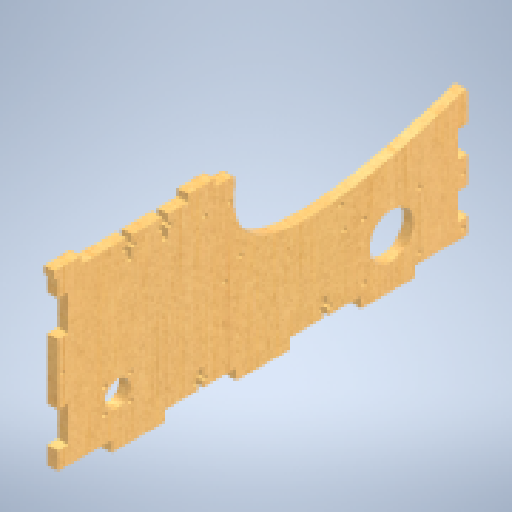
# Autodesk Inventor part: бок
Saved by Autodesk Inventor 2024.2 (Build 282272000, 272)
## iProperties
Created: 2026-01-28
Part Number: бок
Material: Типовые
Document SubType Name: Modeling
Designer: Zakhar
Density: 1 g/cm^3
Appearance: Желтая сосна — массив — светлое морение — со слабым глянцем
Mass: 99.4339 g
Surface Area: 393.183 cm^2
Volume: 99.4339 cm^3
Author: Zakhar
Autodesk Inventor part; units mm, degrees
ref_plane "YZ Plane" through (0, 0, 0) normal (1, 0, 0) x (0, 1, 0)
ref_plane "XZ Plane" through (0, 0, 0) normal (0, 1, 0) x (-1, 0, 0)
ref_plane "XY Plane" through (0, 0, 0) normal (0, 0, 1) x (1, 0, 0)
sketch "Эскиз1" plane through (0, 0, 0) normal (1, 0, 0) x (0, 1, 0)
  line L0 (35.7991, 182.7989) -> (-64.2009, 182.7989)
  line L1 (-64.2009, 182.7989) -> (-64.2009, -47.2011)
  line L2 (-64.2009, -47.2011) -> (35.7991, -47.2011)
  line L3 (35.7991, -47.2011) -> (35.7991, 182.7989)
  spline S0 degree 3 poles (35.7991, 82.7989) (-39.4152, 98.2826) (5.5477, -37.1054) (35.7991, -102.9099) knots 0 0 0 0 1 1 1 1
  line L4 (-4.2009, -47.2011) -> (-19.2009, -47.2011)
  line L5 (-19.2009, -47.2011) -> (-19.2009, -41.2011)
  line L6 (-19.2009, -41.2011) -> (-4.2009, -41.2011)
  line L7 (-4.2009, -41.2011) -> (-4.2009, -47.2011)
  line L8 (-34.2009, -47.2011) -> (-49.2009, -47.2011)
  line L9 (-49.2009, -47.2011) -> (-49.2009, -41.2011)
  line L10 (-49.2009, -41.2011) -> (-34.2009, -41.2011)
  line L11 (-34.2009, -41.2011) -> (-34.2009, -47.2011)
  point P0 (0, 0)
  point P1 (0.0412, 70.0052)
  point P2 (13.562, -47.2011)
  point P3 (-4.2009, -44.2011)
  point P4 (-19.2009, -44.2011)
  point P5 (-34.2009, -44.2011)
  point P6 (-49.2009, -44.2011)
  dimension "d0" = 230
  dimension "d1" = 100
  dimension "d20" = 100
  dimension "d155" = 15
  dimension "d156" = 15
  dimension "d157" = 6
  dimension "d158" = 15
  dimension "d159" = 15
  constraints: 24 end point, 6 parallel, 5 point on line, 4 midpoint, 3 horizontal, 3 perpendicular, 4 other
  measures "d0" distance of L0.end L1.end
  measures "d1" distance of L0.start L0.end
  measures "d20" distance from line of L0 point (35.799, 82.799)
  measures "d155" distance of point (-4.201, -44.201) point (-19.201, -44.201)
  measures "d156" distance of point (-34.201, -44.201) point (-49.201, -44.201)
  measures "d157" distance between parallel lines of L8 L10
  measures "d158" distance of point (-34.201, -44.201) point (-19.201, -44.201)
  measures "d159" distance from line of L1 point (-49.201, -44.201)
extrude "Выдавливание1" add sketch "Эскиз1" along normal blind 6 contours L3 S0 L2 L7 L6 L5 L11 L10 L9 L1 L0
sketch "Эскиз2" plane through (6, 0, 0) normal (1, 0, 0) x (0, 0, -1)
  line L0 (-182.7989, 35.7991) -> (-182.7989, -64.2009) projected
  line L1 (-182.7989, -64.2009) -> (47.2011, -64.2009) projected
  line L2 (-182.7989, -58.2009) -> (-152.7989, -58.2009)
  line L3 (-152.7989, -58.2009) -> (-152.7989, -64.2009)
  line L4 (-152.7989, -64.2009) -> (-182.7989, -64.2009)
  line L5 (-182.7989, -64.2009) -> (-182.7989, -58.2009)
  line L6 (-152.7989, -58.2009) -> (-122.7989, -58.2009)
  line L7 (-122.7989, -58.2009) -> (-122.7989, -64.2009)
  line L8 (-122.7989, -64.2009) -> (-152.7989, -64.2009)
  line L9 (-152.7989, -64.2009) -> (-152.7989, -58.2009)
  line L10 (-122.7989, -58.2009) -> (-82.7989, -58.2009)
  line L11 (-82.7989, -58.2009) -> (-82.7989, -64.2009)
  line L12 (-82.7989, -64.2009) -> (-122.7989, -64.2009)
  line L13 (-122.7989, -64.2009) -> (-122.7989, -58.2009)
  line L14 (47.2011, -64.2009) -> (47.2011, 13.562) projected
  line L15 (47.2011, -58.2009) -> (17.2011, -58.2009)
  line L16 (17.2011, -58.2009) -> (17.2011, -64.2009)
  line L17 (17.2011, -64.2009) -> (47.2011, -64.2009)
  line L18 (47.2011, -64.2009) -> (47.2011, -58.2009)
  line L19 (17.2011, -58.2009) -> (-12.7989, -58.2009)
  line L20 (-12.7989, -58.2009) -> (-12.7989, -64.2009)
  line L21 (-12.7989, -64.2009) -> (17.2011, -64.2009)
  line L22 (17.2011, -64.2009) -> (17.2011, -58.2009)
  line L23 (-12.7989, -58.2009) -> (-52.7989, -58.2009)
  line L24 (-52.7989, -58.2009) -> (-52.7989, -64.2009)
  line L25 (-52.7989, -64.2009) -> (-12.7989, -64.2009)
  line L26 (-12.7989, -64.2009) -> (-12.7989, -58.2009)
  line L27 (-52.7989, -58.2009) -> (-82.7989, -58.2009)
  line L28 (-82.7989, -58.2009) -> (-82.7989, -64.2009)
  line L29 (-82.7989, -64.2009) -> (-52.7989, -64.2009)
  line L30 (-52.7989, -64.2009) -> (-52.7989, -58.2009)
  point P0 (0, 0)
  point P1 (47.89, 35.7991)
  point P2 (-122.7989, -64.2009)
  point P3 (47.2011, 13.562)
  dimension "d4" = 30
  dimension "d5" = 30
  dimension "d6" = 40
  dimension "d7" = 30
  dimension "d8" = 30
  dimension "d9" = 40
  dimension "d12" = 6
  dimension "d13" = 6
  constraints: 56 end point, 14 parallel, 7 horizontal, 7 perpendicular, 7 point on line, 2 other
  measures "d4" distance of L2.start L2.end
  measures "d5" distance of L2.end L6.end
  measures "d6" distance of L6.end L10.end
  measures "d7" distance of L15.start L15.end
  measures "d8" distance of L15.end L19.end
  measures "d9" distance of L19.end L23.end
  measures "d12" distance of L2.end L3.end
  measures "d13" distance of L27.end L11.end
extrude "Выдавливание2" cut sketch "Эскиз2" against normal through all contours L2 L3 L1 L0 | L10 L11 L1 L7 | L23 L20 L1 L24 | L15 L14 L1 L16
sketch "Эскиз3" plane through (0, 0, 0) normal (-1, 0, 0) x (0, 0, 1)
  line L0 (182.7989, -58.2009) -> (176.7989, -58.2009)
  line L1 (176.7989, -58.2009) -> (176.7989, -48.2009)
  line L2 (176.7989, -48.2009) -> (182.7989, -48.2009)
  line L3 (182.7989, -48.2009) -> (182.7989, -58.2009)
  line L4 (176.7989, -48.2009) -> (182.7989, -48.2009)
  line L5 (182.7989, -48.2009) -> (182.7989, -28.2009)
  line L6 (182.7989, -28.2009) -> (176.7989, -28.2009)
  line L7 (176.7989, -28.2009) -> (176.7989, -48.2009)
  line L8 (182.7989, -28.2009) -> (176.7989, -28.2009)
  line L9 (176.7989, -28.2009) -> (176.7989, 5.7991)
  line L10 (176.7989, 5.7991) -> (182.7989, 5.7991)
  line L11 (182.7989, 5.7991) -> (182.7989, -28.2009)
  line L12 (176.7989, 5.7991) -> (182.7989, 5.7991)
  line L13 (182.7989, 5.7991) -> (182.7989, 25.7991)
  line L14 (182.7989, 25.7991) -> (176.7989, 25.7991)
  line L15 (176.7989, 25.7991) -> (176.7989, 5.7991)
  line L16 (182.7989, 35.7991) -> (182.7989, -58.2009) projected
  line L17 (176.7989, 25.7991) -> (182.7989, 25.7991)
  line L18 (182.7989, 25.7991) -> (182.7989, 35.7991)
  line L19 (182.7989, 35.7991) -> (176.7989, 35.7991)
  line L20 (176.7989, 35.7991) -> (176.7989, 25.7991)
  point P0 (0, 0)
  dimension "d14" = 10
  dimension "d15" = 10
  dimension "d16" = 20
  dimension "d17" = 20
  dimension "d106" = 6
  constraints: 40 end point, 10 parallel, 5 horizontal, 5 perpendicular, 3 point on line
  measures "d14" distance of L0.end L1.end
  measures "d15" distance of L19.end L14.end
  measures "d16" distance of L6.end L1.end
  measures "d17" distance of L14.end L9.end
  measures "d106" distance between parallel lines of L16 L15
extrude "Выдавливание3" cut sketch "Эскиз3" against normal blind 6 contours L2 L7 L6 L5 | L10 L15 L14 L13
sketch "Эскиз4" plane through (6, 0, 0) normal (1, 0, 0) x (0, 0, -1)
  line L0 (-16.7989, -58.2009) -> (25.2011, -58.2009)
  line L1 (25.2011, -58.2009) -> (25.2011, -50.2009)
  line L2 (25.2011, -50.2009) -> (-16.7989, -50.2009)
  line L3 (-16.7989, -50.2009) -> (-16.7989, -58.2009)
  line L4 (25.2011, -58.2009) -> (17.2011, -58.2009)
  line L5 (17.2011, -58.2009) -> (17.2011, -16.2009)
  line L6 (17.2011, -16.2009) -> (25.2011, -16.2009)
  line L7 (25.2011, -16.2009) -> (25.2011, -58.2009)
  line L8 (25.2011, -16.2009) -> (-16.7989, -16.2009)
  line L9 (-16.7989, -16.2009) -> (-16.7989, -24.2009)
  line L10 (-16.7989, -24.2009) -> (25.2011, -24.2009)
  line L11 (25.2011, -24.2009) -> (25.2011, -16.2009)
  line L12 (-16.7989, -16.2009) -> (-8.7989, -16.2009)
  line L13 (-8.7989, -16.2009) -> (-8.7989, -58.2009)
  line L14 (-8.7989, -58.2009) -> (-16.7989, -58.2009)
  line L15 (-16.7989, -58.2009) -> (-16.7989, -16.2009)
  line L16 (-16.7989, -45.8935) -> (-16.7989, -53.8935)
  circle A0 centre (-11.2989, -21.7009) radius 1.5
  circle A1 centre (19.7011, -21.7009) radius 1.5
  circle A2 centre (19.7011, -53.2009) radius 1.5
  circle A3 centre (-11.2989, -52.7009) radius 1.5
  circle A4 centre (4.2011, -37.2009) radius 12.5
  line L17 (-182.7989, -58.2009) -> (-152.7989, -58.2009) projected
  line L18 (-176.7989, -28.2009) -> (-176.7989, -48.2009) projected
  circle A5 centre (-149.3429, -37.2009) radius 7
  circle A6 centre (-156.3429, -30.2009) radius 1.5
  circle A7 centre (-142.3429, -30.2009) radius 1.5
  circle A8 centre (-142.3429, -44.2009) radius 1.5
  circle A9 centre (-156.3429, -44.2009) radius 1.5
  line L19 (-142.3429, -30.2009) -> (-142.3429, -44.2009) construction
  line L20 (-142.3429, -44.2009) -> (-156.3429, -44.2009) construction
  line L21 (-156.3429, -30.2009) -> (-156.3429, -44.2009) construction
  line L22 (-156.3429, -30.2009) -> (-142.3429, -30.2009) construction
  line L23 (-67.7989, 21.7334) -> (-67.7989, -91.6472) construction
  line L24 (47.2011, -58.2009) -> (47.2011, 13.562) construction
  line L25 (-152.7989, -64.2009) -> (-122.7989, -64.2009) projected
  point P0 (0, 0)
  point P1 (4.2011, -58.2009)
  point P2 (-176.8137, 14.1065)
  point P3 (-16.7989, -53.8935)
  point P4 (-16.7989, -45.8935)
  point P5 (4.035, -43.7767)
  point P6 (21.9204, -26.629)
  dimension "d21" = 42
  dimension "d22" = 42
  dimension "d23" = 8
  dimension "d24" = 8
  dimension "d25" = 8
  dimension "d26" = 8
  dimension "d27" = 3
  dimension "d28" = 3
  dimension "d29" = 3
  dimension "d30" = 3
  dimension "d31" = 5.5
  dimension "d32" = 5.5
  dimension "d33" = 5.5
  dimension "d34" = 5.5
  dimension "d35" = 5.5
  dimension "d36" = 5.5
  dimension "d37" = 5.5
  dimension "d38" = 21
  dimension "d39" = 21
  dimension "d40" = 25
  dimension "d41" = 3
  dimension "d42" = 160
  dimension "d45" = 14
  dimension "d46" = 3
  dimension "d47" = 3
  dimension "d48" = 3
  dimension "d49" = 3
  dimension "d83" = 115
  dimension "d84" = 27
  constraints: 42 end point, 10 centre point, 9 parallel, 7 perpendicular, 4 horizontal, 4 tangent, 3 vertical, 2 point on line, 1 collinear, 1 midpoint, 3 other
  measures "d21" distance of L10.start L11.start
  measures "d22" distance of L14.end L8.end
  measures "d23" distance between parallel lines of L8 L10
  measures "d24" distance between parallel lines of L7 L5
  measures "d25" distance from line of point (4.201, -58.201) L2
  measures "d26" distance between parallel lines of L15 L13
  measures "d27" diameter of A0
  measures "d28" diameter of A1
  measures "d29" diameter of A2
  measures "d30" diameter of A3
  measures "d31" distance from line of L0 A3.centre
  measures "d32" distance from line of L15 A3.centre
  measures "d33" distance from line of L7 A2.centre
  measures "d34" distance from line of L11 A1.centre
  measures "d35" distance from line of L6 A1.centre
  measures "d36" distance from line of L8 A0.centre
  measures "d37" distance from line of L9 A0.centre
  measures "d38" distance of point (4.201, -58.201) A4.centre
  measures "d39" distance from line of L15 A4.centre
  measures "d40" diameter of A4
  measures "d41" distance from line of L2 A2.centre
  measures "d42" distance between parallel lines of L18 L15
  measures "d45" diameter of A5
  measures "d46" diameter of A6
  measures "d47" diameter of A7
  measures "d48" diameter of A8
  measures "d49" diameter of A9
  measures "d83" distance between parallel lines of L23 L24
  measures "d84" distance from line of L25 A5.centre
extrude "Выдавливание4" cut sketch "Эскиз4" against normal blind 6 contours A0 | A1 | A2 | A3 | A4 | A5 | A6 | A7 | A8 | A9
sketch "Эскиз5" plane through (6, 0, 0) normal (1, 0, 0) x (0, 0, -1)
  line L0 (-82.7989, 35.7991) -> (-182.7989, 35.7991) projected
  line L1 (-144.2989, 35.7991) -> (-141.2989, 35.7991)
  line L2 (-141.2989, 35.7991) -> (-141.2989, 23.7991)
  line L3 (-141.2989, 23.7991) -> (-144.2989, 23.7991)
  line L4 (-144.2989, 23.7991) -> (-144.2989, 35.7991)
  line L5 (-139.2989, 29.3991) -> (-146.2989, 29.3991)
  line L6 (-146.2989, 29.3991) -> (-146.2989, 31.7991)
  line L7 (-146.2989, 31.7991) -> (-139.2989, 31.7991)
  line L8 (-139.2989, 31.7991) -> (-139.2989, 29.3991)
  line L9 (-182.7989, 35.7991) -> (-182.7989, 25.7991) projected
  line L10 (-124.2989, 35.7991) -> (-121.2989, 35.7991)
  line L11 (-121.2989, 35.7991) -> (-121.2989, 23.7991)
  line L12 (-121.2989, 23.7991) -> (-124.2989, 23.7991)
  line L13 (-124.2989, 23.7991) -> (-124.2989, 35.7991)
  line L14 (-119.2989, 29.3991) -> (-126.2989, 29.3991)
  line L15 (-126.2989, 29.3991) -> (-126.2989, 31.7991)
  line L16 (-126.2989, 31.7991) -> (-119.2989, 31.7991)
  line L17 (-119.2989, 31.7991) -> (-119.2989, 29.3991)
  line L18 (-82.7989, 35.7991) -> (-182.7989, 35.7991) projected
  point P0 (0, 0)
  point P1 (-146.2989, 30.5991)
  point P2 (-126.2989, 30.5991)
  point P3 (-121.2989, 29.3991)
  point P4 (-121.2989, 31.7991)
  point P5 (-124.2989, 31.7991)
  point P6 (-124.2989, 29.3991)
  point P7 (-141.2989, 31.7991)
  point P8 (-141.2989, 35.7991)
  point P9 (-144.2989, 31.7991)
  point P10 (-144.2989, 29.3991)
  point P11 (-141.2989, 29.3991)
  point P12 (-182.7989, 30.7991)
  dimension "d50" = 3
  dimension "d51" = 2.4
  dimension "d52" = 7
  dimension "d53" = 2
  dimension "d54" = 12
  dimension "d55" = 4
  dimension "d57" = 3
  dimension "d58" = 2.4
  dimension "d59" = 7
  dimension "d60" = 2
  dimension "d61" = 12
  dimension "d63" = 38.5
  dimension "d66" = 38.5
  constraints: 32 end point, 8 parallel, 4 horizontal, 4 perpendicular, 3 midpoint, 2 collinear, 1 point on line
  measures "d50" distance of L2.end L3.end
  measures "d51" distance between parallel lines of L7 L5
  measures "d52" distance of L6.end L7.end
  measures "d53" distance between parallel lines of L4 L6
  measures "d54" distance of L1.end L2.end
  measures "d55" distance between parallel lines of L0 L7
  measures "d57" distance of L11.end L12.end
  measures "d58" distance between parallel lines of L16 L14
  measures "d59" distance of L15.end L16.end
  measures "d60" distance between parallel lines of L13 L15
  measures "d61" distance of L10.end L11.end
  measures "d63" distance from line of L11 L0.start
  measures "d66" distance from line of point (-182.799, 30.799) L4
extrude "Выдавливание5" cut sketch "Эскиз5" against normal through all
sketch "Эскиз6" plane through (6, 0, 0) normal (1, 0, 0) x (0, 0, -1)
  line L0 (-101.2989, -58.2009) -> (-104.2989, -58.2009)
  line L1 (-104.2989, -58.2009) -> (-104.2989, -48.2009)
  line L2 (-104.2989, -48.2009) -> (-101.2989, -48.2009)
  line L3 (-101.2989, -48.2009) -> (-101.2989, -58.2009)
  line L4 (-106.2989, -52.8009) -> (-99.2989, -52.8009)
  line L5 (-99.2989, -52.8009) -> (-99.2989, -55.2009)
  line L6 (-99.2989, -55.2009) -> (-106.2989, -55.2009)
  line L7 (-106.2989, -55.2009) -> (-106.2989, -52.8009)
  line L8 (-52.7989, -58.2009) -> (-12.7989, -58.2009) projected
  line L9 (-34.2989, -58.2009) -> (-31.2989, -58.2009)
  line L10 (-31.2989, -58.2009) -> (-31.2989, -48.2009)
  line L11 (-31.2989, -48.2009) -> (-34.2989, -48.2009)
  line L12 (-34.2989, -48.2009) -> (-34.2989, -58.2009)
  line L13 (-36.2989, -52.8009) -> (-29.2989, -52.8009)
  line L14 (-29.2989, -52.8009) -> (-29.2989, -55.2009)
  line L15 (-29.2989, -55.2009) -> (-36.2989, -55.2009)
  line L16 (-36.2989, -55.2009) -> (-36.2989, -52.8009)
  line L17 (-122.7989, -58.2009) -> (-82.7989, -58.2009) projected
  line L18 (-122.7989, -64.2009) -> (-122.7989, -58.2009) projected
  line L19 (-52.7989, -64.2009) -> (-52.7989, -58.2009) projected
  point P0 (0, 0)
  point P1 (-122.7989, -61.2009)
  point P2 (-29.2989, -54.0009)
  point P3 (-32.7989, -58.2009)
  point P4 (-34.2989, -55.2009)
  point P5 (-31.2989, -55.2009)
  point P6 (-31.2989, -52.8009)
  point P7 (-34.2989, -52.8009)
  point P8 (-104.2989, -55.2009)
  point P9 (-101.2989, -55.2009)
  point P10 (-101.2989, -52.8009)
  point P11 (-104.2989, -52.8009)
  dimension "d67" = 10
  dimension "d68" = 2.4
  dimension "d69" = 3
  dimension "d70" = 7
  dimension "d71" = 3
  dimension "d72" = 2
  dimension "d73" = 18.5
  dimension "d74" = 3
  dimension "d75" = 10
  dimension "d76" = 2.4
  dimension "d77" = 7
  dimension "d78" = 2
  dimension "d79" = 3
  dimension "d80" = 18.5
  constraints: 32 end point, 8 parallel, 4 horizontal, 4 perpendicular, 3 midpoint, 1 collinear, 1 point on line
  measures "d67" distance of L2.end L0.start
  measures "d68" distance between parallel lines of L6 L4
  measures "d69" distance between parallel lines of L0 L6
  measures "d70" distance of L5.end L6.end
  measures "d71" distance between parallel lines of L1 L3
  measures "d72" distance between parallel lines of L7 L1
  measures "d73" distance from line of point (-122.799, -61.201) L1
  measures "d74" distance of L10.end L11.end
  measures "d75" distance of L9.end L10.end
  measures "d76" distance of L13.end L14.end
  measures "d77" distance of L14.end L15.end
  measures "d78" distance from line of L10 point (-29.299, -54.001)
  measures "d79" distance from line of point (-32.799, -58.201) L15
  measures "d80" distance between parallel lines of L19 L12
extrude "Выдавливание6" cut sketch "Эскиз6" against normal through all
sketch "Эскиз7" plane through (6, 0, 0) normal (1, 0, 0) x (0, 0, -1)
  line L0 (-182.7989, 35.7991) -> (-214.7989, 35.7991)
  line L1 (-214.7989, 35.7991) -> (-214.7989, -58.2009)
  line L2 (-214.7989, -58.2009) -> (-182.7989, -58.2009)
  line L3 (-182.7989, -58.2009) -> (-182.7989, 35.7991)
  line L4 (-182.7989, -58.2009) -> (-152.7989, -58.2009) projected
  line L5 (-182.7989, -48.2009) -> (-182.7989, -58.2009) projected
  line L6 (-144.2989, 35.7991) -> (-182.7989, 35.7991) projected
  point P0 (0, 0)
  dimension "d85" = 32
  constraints: 8 end point, 3 collinear, 2 parallel, 1 horizontal, 1 perpendicular
  measures "d85" distance of L1.end L2.end
extrude "Выдавливание7" [suppressed]
sketch "Эскиз8" plane through (6, 0, 0) normal (1, 0, 0) x (0, 0, -1)
  circle A0 centre (-212.7989, -19.2009) radius 1.5
  circle A1 centre (-186.7989, -19.2009) radius 1.5
  circle A2 centre (-186.7989, -45.2009) radius 1.5
  circle A3 centre (-212.7989, -45.2009) radius 1.5
  line L0 (-182.7989, 5.7991) -> (-182.7989, 25.7991) projected
  line L1 (-144.2989, 35.7991) -> (-182.7989, 35.7991) projected
  line L2 (-214.7989, -58.2009) -> (-152.7989, -58.2009) projected
  circle A4 centre (-199.7989, -32.2009) radius 7
  point P0 (0, 0)
  point P1 (-214.7989, 35.7991)
  dimension "d92" = 3
  dimension "d93" = 26
  dimension "d98" = 4
  dimension "d99" = 4
  dimension "d104" = 13
  dimension "d105" = 13
  dimension "d116" = 14
  dimension "d139" = 13
  dimension "d140" = 13
  dimension "d141" = 13
  dimension "d142" = 13
  dimension "d143" = 13
  constraints: 5 centre point, 3 equal radius
  measures "d92" diameter of A2
  measures "d93" distance of A2.centre A1.centre
  measures "d98" distance from line of L0 A2.centre
  measures "d99" distance from line of L0 A1.centre
  measures "d104" distance from line of L2 A2.centre
  measures "d105" distance from line of L2 A3.centre
  measures "d116" diameter of A4
  measures "d139" horizontal distance of A0.centre A4.centre
  measures "d140" horizontal distance of A1.centre A4.centre
  measures "d141" horizontal distance of A3.centre A4.centre
  measures "d142" horizontal distance of A3.centre A4.centre
  measures "d143" horizontal distance of A0.centre A4.centre
extrude "Выдавливание8" cut sketch "Эскиз8" against normal through all
sketch "Эскиз9" plane through (0, 0, 0) normal (-1, 0, 0) x (0, 0, 1)
  line L0 (144.2989, 35.7991) -> (182.7989, 35.7991) projected
  line L1 (188.2989, 35.7991) -> (191.2989, 35.7991)
  line L2 (191.2989, 35.7991) -> (191.2989, 25.7991)
  line L3 (191.2989, 25.7991) -> (188.2989, 25.7991)
  line L4 (188.2989, 25.7991) -> (188.2989, 35.7991)
  line L5 (193.2989, 31.3991) -> (186.2989, 31.3991)
  line L6 (186.2989, 31.3991) -> (186.2989, 33.7991)
  line L7 (186.2989, 33.7991) -> (193.2989, 33.7991)
  line L8 (193.2989, 33.7991) -> (193.2989, 31.3991)
  line L9 (214.7989, -58.2009) -> (214.7989, 35.7991) projected
  point P0 (0, 0)
  point P1 (188.2989, 31.3991)
  point P2 (191.2989, 31.3991)
  point P3 (191.2989, 33.7991)
  point P4 (188.2989, 33.7991)
  dimension "d107" = 3
  dimension "d108" = 23.5
  dimension "d109" = 7
  dimension "d110" = 2
  dimension "d111" = 10
  dimension "d112" = 2.4
  dimension "d113" = 2
  constraints: 16 end point, 4 parallel, 2 horizontal, 2 perpendicular, 1 point on line
  measures "d107" distance between parallel lines of L4 L2
  measures "d108" distance between parallel lines of L9 L2
  measures "d109" distance of L5.start L5.end
  measures "d110" distance between parallel lines of L2 L8
  measures "d111" distance of L1.end L2.end
  measures "d112" distance between parallel lines of L7 L5
  measures "d113" distance between parallel lines of L0 L7
extrude "Выдавливание9" cut sketch "Эскиз9" against normal blind 10
fillet "Сопряжение1" radius 2 2 edges at (3, 35.7991, 82.7989) (3, 13.562, -47.2011)
sketch "Эскиз11" plane through (0, 0, 0) normal (-1, 0, 0) x (0, 0, 1)
  circle A0 centre (100.1841, 23.904) radius 1.5
  circle A1 centre (89.0971, -13.4435) radius 1.5
  circle A2 centre (23.5119, -8.8427) radius 1.5
  circle A3 centre (86.4418, 23.904) radius 1.5
  circle A4 centre (80.5036, -4.7593) radius 1.5
  circle A5 centre (22.0119, -21.3866) radius 1.5
  point P0 (0, 0)
  dimension "d134" = 3
  dimension "d135" = 3
  dimension "d136" = 3
  dimension "d144" = 3
  dimension "d145" = 3
  dimension "d146" = 3
  constraints: 6 centre point
  measures "d134" diameter of A2
  measures "d135" diameter of A1
  measures "d136" diameter of A0
  measures "d144" diameter of A3
  measures "d145" diameter of A4
  measures "d146" diameter of A5
extrude "Выдавливание11" cut sketch "Эскиз11" against normal blind 10
sketch "Эскиз12" plane through (0, 0, 0) normal (-1, 0, 0) x (0, 0, 1)
  line L0 (144.2989, 35.7991) -> (182.7989, 35.7991) projected
  line L1 (184.7989, 35.7991) -> (169.7989, 35.7991)
  line L2 (169.7989, 35.7991) -> (169.7989, 39.7991)
  line L3 (169.7989, 39.7991) -> (184.7989, 39.7991)
  line L4 (184.7989, 39.7991) -> (184.7989, 35.7991)
  line L5 (214.7989, -58.2009) -> (214.7989, 35.7991) projected
  line L6 (109.7989, 35.7991) -> (94.7989, 35.7991)
  line L7 (94.7989, 35.7991) -> (94.7989, 39.7991)
  line L8 (94.7989, 39.7991) -> (109.7989, 39.7991)
  line L9 (109.7989, 39.7991) -> (109.7989, 35.7991)
  line L10 (214.7989, 35.7991) -> (84.7989, 35.7991) projected
  line L11 (85.2096, 35.7991) -> (121.2989, 35.7991) projected
  point P0 (0, 0)
  point P1 (188.2989, 35.7991)
  point P2 (184.7989, 37.7991)
  point P3 (169.7989, 37.7991)
  point P4 (109.7989, 37.7991)
  point P5 (94.7989, 37.7991)
  dimension "d147" = 4
  dimension "d148" = 30
  dimension "d149" = 15
  dimension "d150" = 4
  dimension "d151" = 60
  dimension "d152" = 15
  constraints: 16 end point, 4 midpoint, 4 parallel, 2 horizontal, 2 perpendicular, 1 collinear, 1 point on line
  measures "d147" distance of L3.end L1.start
  measures "d148" distance between parallel lines of L5 L4
  measures "d149" distance of point (184.799, 37.799) point (169.799, 37.799)
  measures "d150" distance of L8.end L6.start
  measures "d151" distance of point (169.799, 37.799) point (109.799, 37.799)
  measures "d152" distance of point (94.799, 37.799) point (109.799, 37.799)
extrude "Выдавливание12" add sketch "Эскиз12" against normal blind 6
sketch "Эскиз13" plane through (6, 0, 0) normal (1, 0, 0) x (0, 0, -1)
  circle A0 centre (44.2011, -26.7009) radius 1.5
  circle A1 centre (44.2011, -53.7009) radius 1.5
  line L0 (41.2011, -34.2009) -> (47.2011, -34.2009) projected
  line L1 (47.2011, -34.2009) -> (47.2011, -19.2009) projected
  line L2 (47.2011, -49.2009) -> (41.2011, -49.2009) projected
  line L3 (47.2011, -58.2009) -> (47.2011, -49.2009) projected
  circle A2 centre (-179.7989, -12.2009) radius 1.5
  line L4 (-152.7989, -64.2009) -> (-122.7989, -64.2009) projected
  line L5 (-176.7989, -28.2009) -> (-176.7989, -48.2009) projected
  point P0 (0, 0)
  point P1 (44.2011, -34.2009)
  point P2 (44.2011, -49.2009)
  dimension "d160" = 3
  dimension "d161" = 3
  dimension "d162" = 7.5
  dimension "d163" = 3
  dimension "d164" = 4.5
  dimension "d165" = 3
  dimension "d168" = 3
  dimension "d169" = 52
  dimension "d170" = 3
  constraints: 3 centre point, 2 midpoint
  measures "d160" diameter of A0
  measures "d161" diameter of A1
  measures "d162" distance of point (44.201, -34.201) A0.centre
  measures "d163" distance from line of L1 A0.centre
  measures "d164" distance of point (44.201, -49.201) A1.centre
  measures "d165" distance from line of L3 A1.centre
  measures "d168" diameter of A2
  measures "d169" distance from line of L4 A2.centre
  measures "d170" distance from line of A2.centre L5
extrude "Выдавливание13" cut sketch "Эскиз13" against normal blind 6
sketch "Эскиз14" plane through (6, 0, 0) normal (1, 0, 0) x (0, 0, -1)
  line L0 (-199.1415, 35.7991) -> (-199.1415, -19.3906)
  line L1 (-82.7989, 35.7991) -> (-121.2989, 35.7991) projected
  line L2 (-214.7989, 35.7991) -> (-214.7989, -58.2009) projected
  circle A0 centre (-199.7989, -32.2009) radius 7 projected
  line L3 (-214.7989, -58.2009) -> (-152.7989, -58.2009) projected
  line L4 (-199.1415, -19.3906) -> (-214.7989, -32.2009)
  line L5 (-197.5588, -58.2009) -> (-214.7989, -32.2009)
  line L6 (-182.7989, 10.2991) -> (-186.7989, 10.2991)
  line L7 (-186.7989, 10.2991) -> (-186.7989, 1.2991)
  line L8 (-186.7989, 1.2991) -> (-182.7989, 1.2991)
  line L9 (-182.7989, 1.2991) -> (-182.7989, 10.2991)
  line L10 (-182.7989, 5.7991) -> (-182.7989, 25.7991) projected
  line L11 (-192.7989, 15.7991) -> (-184.7989, 15.7991)
  line L12 (-184.7989, 15.7991) -> (-184.7989, -4.2009)
  line L13 (-184.7989, -4.2009) -> (-192.7989, -4.2009)
  line L14 (-192.7989, -4.2009) -> (-192.7989, 15.7991)
  point P0 (0, 0)
  point P1 (-191.2989, 35.7991)
  point P2 (-184.7989, 10.2991)
  point P3 (-188.7989, -4.2009)
  point P4 (-184.7989, 10.2991)
  point P5 (-184.7989, 1.2991)
  dimension "d171" = 25.5
  dimension "d172" = 9
  dimension "d173" = 4
  dimension "d174" = 5.5
  dimension "d175" = 20
  dimension "d176" = 8
  dimension "d177" = 2
  constraints: 22 end point, 4 parallel, 2 horizontal, 2 midpoint, 2 perpendicular, 2 point on line, 1 collinear, 1 vertical
  measures "d171" distance from line of L1 point (-184.799, 10.299)
  measures "d172" distance of L6.end L7.end
  measures "d173" distance of L7.end L8.end
  measures "d174" distance from line of L8 point (-188.799, -4.201)
  measures "d175" distance of L13.end L11.start
  measures "d176" distance of L11.start L11.end
  measures "d177" distance between parallel lines of L9 L12
extrude "Выдавливание14" [suppressed]
sketch "Эскиз10" plane through (6, 0, 0) normal (1, 0, 0) x (0, 0, -1)
  circle A0 centre (-170.61, 18.2991) radius 1.5
  circle A1 centre (-139.61, 18.2991) radius 1.5
  circle A2 centre (-139.61, -12.7009) radius 1.5
  circle A3 centre (-170.61, -12.7009) radius 1.5
  line L0 (-176.7989, 25.7991) -> (-176.7989, 5.7991) projected
  line L1 (-144.2989, 35.7991) -> (-188.2989, 35.7991) projected
  point P0 (0, 0)
  dimension "d119" = 3
  dimension "d120" = 3
  dimension "d121" = 3
  dimension "d122" = 3
  dimension "d123" = 5.5
  dimension "d124" = 17.5
  dimension "d125" = 17.5
  dimension "d126" = 31
  dimension "d127" = 0
  dimension "d128" = 31
  dimension "d129" = 0
  dimension "d130" = 31
  constraints: 4 centre point
  measures "d119" diameter of A0
  measures "d120" diameter of A1
  measures "d121" diameter of A2
  measures "d122" diameter of A3
  measures "d124" distance from line of L1 A0.centre
  measures "d125" distance from line of L1 A1.centre
  measures "d126" distance of A0.centre A1.centre
  measures "d127" horizontal distance of A3.centre A0.centre
  measures "d128" distance of A0.centre A3.centre
  measures "d129" horizontal distance of A1.centre A2.centre
  measures "d130" distance of A1.centre A2.centre
equation "\"d28\" = d27"
equation "\"d29\" = d27"
equation "\"d30\" = d27"
